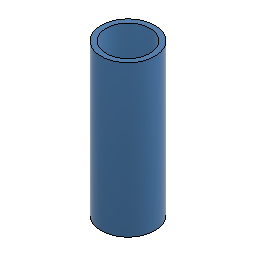
fluke_bracket_1_asm (Autodesk Fusion 360 archive; units mm, degrees)
design "probeHolder4040"
Autodesk Fusion 360 part; units mm, degrees
sketch "Sketch1" plane through (0, 0, 0) normal (0, 1, 0) x (1, 0, 0)
  circle A0 centre (0, 0) radius 13
  circle A1 centre (0, 0) radius 16
  circle A2 centre (0, 0) radius 4.25
  dimension "d1" = 26
  dimension "d2" = 32
  dimension "d3" = 8.5
  constraint coincident A0.centre A1.centre
  constraint concentric A0 A2
  measures "d1" diameter of A0
  measures "d2" diameter of A1
  measures "d3" diameter of A2
extrude "Extrude1" add sketch "Sketch1" along normal blind 4 contours A0 | A1
extrude "Extrude2" add sketch "Sketch1" along normal blind 90 contours A1

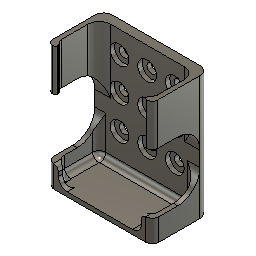
design "fluke_bracket_1"
Autodesk Fusion 360 part; units mm, degrees
sketch "Sketch1" plane through (0, 0, 0) normal (0, 0, 1) x (1, 0, 0)
  line L0 (47.5, 56) -> (-47.5, 56)
  line L1 (-47.5, 56) -> (-47.5, -56)
  line L2 (-47.5, -56) -> (47.5, -56)
  line L3 (47.5, -56) -> (47.5, 56)
  line L4 (47.5, 56) -> (-47.5, -56) construction
  line L5 (-47.5, 56) -> (47.5, -56) construction
  line L6 (-43.5, 56) -> (-43.5, -52)
  line L7 (-43.5, -52) -> (47.5, -52)
  line L8 (43.5, -52) -> (43.5, 56)
  line L9 (43.5, 52) -> (-43.5, -52) construction
  line L10 (-43.5, 52) -> (43.5, -52) construction
  line L11 (-43.5, -52) -> (-43.5, -56)
  line L12 (43.5, -52) -> (43.5, -56)
  line L13 (-43.5, -52) -> (-47.5, -52)
  circle A0 centre (-0.166, 36) radius 4.25
  circle A1 centre (-25.166, 36) radius 4.25
  circle A2 centre (24.834, 36) radius 4.25
  line L14 (-43.5, -50.9745) -> (43.5, -50.9745)
  line L15 (-39.9513, -50.9745) -> (-39.9513, -52)
  circle A3 centre (-25.166, 6) radius 4.25
  circle A4 centre (-0.166, 6) radius 4.25
  circle A5 centre (24.834, 6) radius 4.25
  circle A6 centre (-25.166, -24) radius 4.25
  circle A7 centre (-0.166, -24) radius 4.25
  circle A8 centre (24.834, -24) radius 4.25
  circle A9 centre (-25.166, 36) radius 8.5
  circle A10 centre (-25, 36) radius 7.5
  circle A11 centre (-0.166, 36) radius 8.5
  circle A12 centre (24.834, 36) radius 8.5
  circle A13 centre (-25.166, 6) radius 8.5
  circle A14 centre (-0.166, 6) radius 8.5
  circle A15 centre (24.834, 6) radius 8.5
  circle A16 centre (-25.166, -24) radius 8.5
  circle A17 centre (-0.166, -24) radius 8.5
  circle A18 centre (24.834, -24) radius 8.5
  line L16 (-105, 19) -> (-67, 19) construction
  line L17 (-67, 19) -> (-67, 30) construction
  line L18 (-67, 30) -> (-105, 30) construction
  line L19 (-105, 30) -> (-105, 19) construction
  dimension "d1" = 95
  dimension "d2" = 112
  dimension "d7" = 4
  dimension "d8" = 4
  dimension "d9" = 4
  dimension "d48" = 8.5
  dimension "d49" = 20
  dimension "d50" = 8.5
  dimension "d51" = 25
  dimension "d52" = 8.5
  dimension "d53" = 25
  dimension "d83" = 0
  dimension "d84" = -60
  dimension "d99" = 17
  dimension "d100" = 15
  dimension "d103" = 50
  dimension "d104" = -60
  dimension "d134" = 20
  dimension "d135" = 20
  dimension "d136" = 20
  dimension "d161" = 10
  constraint horizontal L0
  constraint perpendicular L0 L1
  constraint parallel L0 L2
  constraint parallel L1 L3
  constraint coincident L4 origin
  constraint coincident L5 origin
  constraint parallel L6 L8
  constraint coincident L9 origin
  constraint coincident L10 origin
  constraint coincident L0 L6.start
  constraint coincident L10.start L6
  constraint coincident L0 L8.end
  constraint coincident L9.start L8
  constraint coincident L2 L11.end
  constraint perpendicular L2 L11
  constraint coincident L2 L12.end
  constraint perpendicular L2 L12
  constraint coincident L1 L13.end
  constraint perpendicular L1 L13
  constraint coincident L8.start L7
  constraint coincident L3 L7.end
  constraint coincident L6 L14.start
  constraint coincident L8 L14.end
  constraint perpendicular L8 L14
  constraint coincident L14 L15.start
  constraint coincident L7 L15.end
  constraint perpendicular L7 L15
  constraint concentric A1 A9
  measures "d1" distance of L1.end L2.end
  measures "d2" distance of L0.end L1.end
  measures "d7" distance of L2 L7
  measures "d8" distance of L1 L6
  measures "d9" distance of L3 L8
  measures "d48" diameter of A0
  measures "d49" distance of L0 A0.centre
  measures "d50" diameter of A1
  measures "d51" distance of A0.centre A1.centre
  measures "d52" diameter of A2
  measures "d53" distance of A0.centre A2.centre
  measures "d99" diameter of A9
  measures "d100" diameter of A10
  measures "d134" distance of L0 A1.centre
  measures "d135" distance of L0 A2.centre
  measures "d136" distance of L0 A10.centre
extrude "Extrude1" add sketch "Sketch1" along normal blind 8 contours L0 L3 L7 L8 | L0 L6 L8 L14 | L2 L3 L7 L12 | L0 L1 L6 L13 | L7 L8 L14 L15 | L2 L7 L11 L12 | L6 L7 L14 L15 | L1 L2 L11 L13 | A0 | A1 | A2 | A3 | A4 | A5 | A6 | A7 | A8 | A9 | A10 | A11 | A12 | A13 | A14 | A15 | A16 | A17 | A18
extrude "Extrude2" add sketch "Sketch1" along normal blind 51 contours L2 L3 L7 L12 | L2 L7 L11 L12 | L1 L2 L11 L13
sketch "Sketch2" plane through (0, 0, 0) normal (0, 1, 0) x (1, 0, 0)
  line L0 (-47.5, 0) -> (-47.5, -51)
  line L1 (-47.5, -51) -> (-37.5, -51)
  line L2 (-37.5, -51) -> (-37.5, -47)
  line L3 (-37.5, -47) -> (-43.5, -47)
  line L4 (-43.5, -47) -> (-43.5, 0)
  line L5 (-43.5, 0) -> (-47.5, 0)
  line L6 (47.5, 0) -> (-47.5, 0)
  line L7 (47.5, 0) -> (47.5, -51)
  line L8 (47.5, -51) -> (37.5, -51)
  line L9 (37.5, -51) -> (37.5, -47)
  line L10 (37.5, -47) -> (43.5, -47)
  line L11 (43.5, -47) -> (43.5, 0)
  line L12 (-40.5, -51) -> (-47.5, -51)
  line L13 (-40.5, -51) -> (-40.5, -47)
  line L14 (-40.5, -47) -> (-47.5, -47)
  line L15 (-47.5, 0) -> (47.5, 0)
  line L16 (40.5, -51) -> (47.5, -51)
  line L17 (40.5, -51) -> (40.5, -47)
  line L18 (40.5, -47) -> (47.5, -47)
  point P0 (-0.166, 0)
  dimension "d16" = 4
  dimension "d17" = 47
  dimension "d18" = 4
  dimension "d19" = 10
  dimension "d64" = 10
  dimension "d65" = 4
  dimension "d66" = 4
  dimension "d89" = 47
  dimension "d121" = 4
  dimension "d122" = 47
  dimension "d123" = 7
  dimension "d125" = 7
  dimension "d132" = 47
  dimension "d133" = 4
  constraint vertical L0
  constraint perpendicular L0 L1
  constraint perpendicular L1 L2
  constraint perpendicular L2 L3
  constraint perpendicular L3 L4
  constraint perpendicular L4 L5
  constraint coincident L4.end L6
  constraint coincident L6.start L7.start
  constraint perpendicular L6 L7
  constraint perpendicular L7 L8
  constraint perpendicular L3 L9
  constraint perpendicular L2 L10
  constraint coincident L6 L11.end
  constraint perpendicular L6 L11
  constraint coincident L0 L1.start
  constraint perpendicular L0 L12
  constraint perpendicular L12 L13
  constraint coincident L0 L14.end
  constraint perpendicular L0 L14
  constraint coincident L7 L8.start
  constraint perpendicular L7 L16
  constraint perpendicular L14 L17
  constraint coincident L7 L18.end
  constraint perpendicular L7 L18
  constraint coincident L0.start L5.end
  measures "d16" distance of L1 L3
  measures "d17" distance of L3 L6
  measures "d18" distance of L0 L4
  measures "d19" distance of L0.end L1.end
  measures "d64" distance of L7.end L8.end
  measures "d65" distance of L7 L11
  measures "d66" distance of L8 L10
  measures "d89" distance of L6 L10
  measures "d121" distance of L12.start L13.end
  measures "d122" distance of L14 L15
  measures "d123" distance of L12.start L0.end
  measures "d125" distance of L7 L16.start
  measures "d132" distance of L6 L18
  measures "d133" distance of L16 L18
extrude "Extrude3" add sketch "Sketch2" along normal blind 18 and the other way blind -56 contours L0 L4 L5 L6 L14 L15 | L0 L1 L3 L12 L13 L14 | L6 L7 L11 L15 L18 | L7 L8 L10 L16 L17 L18
extrude "Extrude4" add sketch "Sketch2" along normal blind -55 and the other way blind 36
fillet "Fillet3" radius 10.5 1 edges at (-43.5, 37, 8)
fillet "Fillet4" radius 6 1 edges at (-47.5, -46, 51)
fillet "Fillet5" radius 8 1 edges at (-43.5, -44, 47)
fillet "Fillet6" radius 6 1 edges at (-43.5, -44, 8)
fillet "Fillet12" radius 20 1 edges at (-40.25, 18, 8)
extrude "Extrude5" cut sketch "Sketch1" along normal blind 12 contours A0 | A1 | A2 | A3 | A4 | A5 | A6 | A7 | A8
fillet "Fillet16" radius 10 1 edges at (43.5, 37, 8)
extrude "Extrude7" cut sketch "Sketch1" along normal blind 8 and the other way blind -4 contours A9 | A10 | A11 | A12 | A13 | A14 | A15 | A16 | A17 | A18
fillet "Fillet29" radius 4.5 1 edges at (-37.5, -36, 49)
fillet "Fillet32" radius 4 1 edges at (37.5, -36, 49)
fillet "Fillet33" radius 5 1 edges at (43.5, -44, 47)
fillet "Fillet35" radius 5.5 2 edges at (-43.5, 37, 47) (43.5, 37, 47)
fillet "Fillet36" radius 5 2 edges at (-47.5, 37, 51) (47.5, 37, 51)
fillet "Fillet37" radius 2 4 edges at (-40.5, 37, 47) (-40.5, 37, 51) (40.5, 37, 47) (40.5, 37, 51)
fillet "Fillet38" radius 8 2 edges at (47.5, 0, 0) (-47.5, 0, 0)
fillet "Fillet39" radius 20 2 edges at (-42.5, -36, 8) (45.5, -36, 8)
fillet "Fillet40" radius 7.5 1 edges at (43.5, -34, 8)
fillet "Fillet41" radius 5.5 8 edges at (38, -52, 47) (42.0355, -52, 45.5355) (43.5, -52, 28.75) (41.3033, -52, 10.1967) (-0.75, -52, 8) (-41.7426, -52, 9.7574) (-43.5, -52, 26.627) (-41.8246, -52, 44.153)
fillet "Fillet42" radius 8 2 edges at (-37.5, -52, 45.877) (37.5, -52, 46.25)
fillet "Fillet43" radius 20.5 1 edges at (40.5, 18, 8)
fillet "Fillet44" radius 6 1 edges at (47.5, -46, 51)
equation "d1 = WidthInternal + WidthSide + WidthSide"
equation "d2 = Height"
equation "d16 = LowLipThickness"
equation "d17 = LowDepth"
equation "d18 = WidthSide"
equation "d19 = LowLip"
equation "d64 = LowLip"
equation "d65 = WidthSide"
equation "d66 = LowLipThickness"
equation "d89 = LowDepth"
equation "d121 = UpperLipThickness"
equation "d122 = UpperDepth"
equation "d123 = UpperLip"
equation "d125 = UpperLip"
equation "d132 = UpperDepth"
equation "d133 = UpperLipThickness"
equation "UpperDepth = 47 mm" comment "30=fluke77 & fluke26, 22=fluke8060A, 47=LCRmeter,"
equation "LowDepth = 47 mm"
equation "UpperLip = 7 mm"
equation "LowLip = 10 mm"
equation "WidthSide = 4 mm"
equation "UpperLipThickness = 4 mm"
equation "LowLipThickness = 4 mm"
equation "Width = 95 mm"
equation "Height = 112 mm"
equation "WidthInternal = 87 mm"

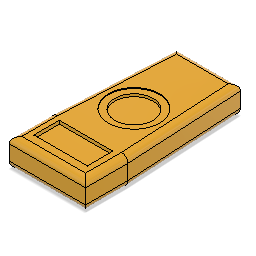
design "fluke_26"
Autodesk Fusion 360 part; units mm, degrees
sketch "Sketch1" plane through (0, 0, 0) normal (0, 1, 0) x (1, 0, 0)
  line L0 (-37.5, -95) -> (37.5, -95)
  line L1 (37.5, -95) -> (37.5, 95)
  line L2 (37.5, 95) -> (-37.5, 95)
  line L3 (-37.5, 95) -> (-37.5, -95)
  line L4 (-37.5, -95) -> (37.5, 95) construction
  line L5 (37.5, -95) -> (-37.5, 95) construction
  line L6 (-45, -95) -> (45, -95)
  line L7 (45, -95) -> (45, 95)
  line L8 (45, 95) -> (-45, 95)
  line L9 (-45, 95) -> (-45, -95)
  line L10 (-45, -95) -> (45, 95) construction
  line L11 (45, -95) -> (-45, 95) construction
  line L12 (45, -45) -> (-45, -45)
  line L13 (45, -45) -> (37.5, 95)
  line L14 (-45, -45) -> (-37.5, 95)
  line L15 (31.1842, -79) -> (-31.8158, -79)
  line L16 (-31.8158, -79) -> (-31.8158, -49)
  line L17 (-31.8158, -49) -> (31.1842, -49)
  line L18 (31.1842, -49) -> (31.1842, -79)
  circle A0 centre (0, 7) radius 22.5
  circle A1 centre (0, 7) radius 30
  dimension "d1" = 75
  dimension "d2" = 190
  dimension "d3" = 190
  dimension "d4" = 50
  dimension "d5" = 63
  dimension "d6" = 30
  dimension "d7" = 16
  dimension "d16" = 45
  dimension "d17" = 88
  dimension "d18" = 60
  constraint horizontal L0
  constraint perpendicular L0 L1
  constraint parallel L0 L2
  constraint parallel L1 L3
  constraint coincident L4 origin
  constraint coincident L5 origin
  constraint horizontal L6
  constraint perpendicular L6 L7
  constraint parallel L6 L8
  constraint parallel L7 L9
  constraint coincident L10 origin
  constraint coincident L11 origin
  constraint coincident L7 L12.start
  constraint coincident L9 L12.end
  constraint perpendicular L9 L12
  constraint horizontal L15
  constraint vertical L16
  constraint horizontal L17
  constraint vertical L18
  constraint coincident L5 L15.start
  constraint concentric A0 A1
  measures "d1" distance of L1.end L2.end
  measures "d2" distance of L0.end L1.end
  measures "d3" distance of L6.end L7.end
  measures "d4" distance of L0 L12
  measures "d5" distance of L15.start L15.end
  measures "d6" distance of L15.start L17.end
  measures "d7" distance of L6 L15
  measures "d16" diameter of A0
  measures "d17" distance of L2 A0.centre
  measures "d18" diameter of A1
extrude "Extrude1" add sketch "Sketch1" against normal blind 33 contours L0 L1 L3 L6 L12 | L3 L6 L9 L12 | L1 L6 L7 L12 | L3 L12 L14 | L1 L2 L3 L8 L12 | L1 L12 L13 | L15 L16 L17 L18 | A0 | A1
extrude "Extrude2" cut sketch "Sketch1" against normal blind 4 contours L15 L16 L17 L18 | A0
fillet "Fillet1" radius 7.5 6 edges at (45, 0, 70) (41.25, 0, -25) (0, 0, 95) (-45, 0, 70) (-41.25, 0, -25) (0, 0, -95)
fillet "Fillet2" radius 8 6 edges at (0, -33, 95) (45, -33, 70) (41.25, -33, -25) (0, -33, -95) (-41.25, -33, -25) (-45, -33, 70)
extrude "Extrude3" cut sketch "Sketch1" against normal blind 1 contours A1
